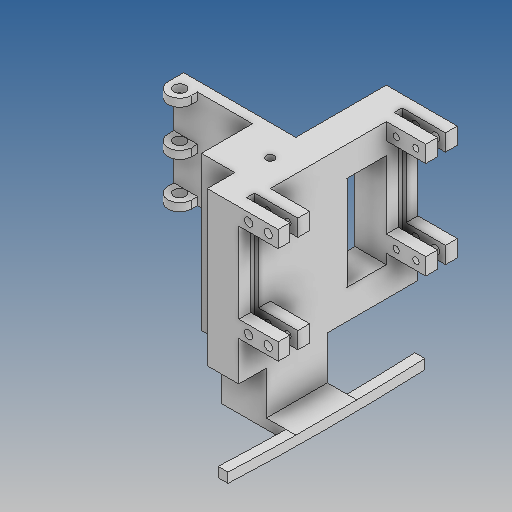
# Autodesk Inventor part: Korpus
Saved by Autodesk Inventor 2026.2 (Build 302298000, 298)
## iProperties
Created: 2025-08-31
Part Number: Korpus
Material: Generisch
Document SubType Name: Modeling
Designer: weyer
Density: 1 g/cm^3
Appearance: Vorgabe
Author: weyer
Autodesk Inventor part; units mm, degrees
sketch "Skizze1" plane through (0, 0, 0) normal (0, 0, 1) x (1, 0, 0)
  line L0 (-9.5, -10.5) -> (7.5, -10.5)
  line L1 (7.5, -10.5) -> (7.5, 10.5)
  line L2 (7.5, 10.5) -> (-9.5, 10.5)
  line L3 (-14.1, 0) -> (18.1, 0) projected
  line L4 (0, -21.7) -> (0, 21.7) projected
  line L5 (-9.5, -10.5) -> (-9.5, -15.5)
  line L6 (-9.5, -15.5) -> (13.5, -15.5)
  line L7 (-9.5, 10.5) -> (-9.5, 15.5)
  line L8 (-9.5, 15.5) -> (13.5, 15.5)
  line L9 (13.5, 15.5) -> (13.5, -15.5)
  point P0 (0, 0)
  dimension "d2" = 21
  dimension "d4" = 7.5
  dimension "d5" = 5
  dimension "d8" = 5
  dimension "d9" = 23
  dimension "d147" = 6
  dimension "d148" = 23
  constraints: 16 end point, 4 perpendicular, 2 vertical, 1 horizontal, 1 other
  measures "d2" distance between parallel lines of L0 L2
  measures "d4" distance between parallel lines of L1 L4
  measures "d5" distance of L0.start L5.end
  measures "d8" distance of L2.end L7.end
  measures "d9" distance of L7.end L8.end
  measures "d147" distance between parallel lines of L1 L9
  measures "d148" distance between parallel lines of L9 L5
extrude "Tower" add sketch "Skizze1" against normal blind 95 contours L0 L4 L6 L5 | L0 L1 L3 L9 L6 L4 | L1 L2 L4 L8 L9 L3 | L2 L7 L8 L4
ref_plane "Arbeitsebene1" through (0, 0, -95) normal (0, 0, -1) x (-1, 0, 0)
sketch "Skizze6" plane through (-9.5, 15.5, 0) normal (0, 1, 0) x (1, 0, 0)
  line L0 (23, 0) -> (23, 95) projected
  line L1 (23, 66.4131) -> (23, 0)
  line L2 (246, -7) -> (246, -5)
  line L3 (0, 0) -> (0, 95) projected
  line L4 (0, 0) -> (23, 0) projected
  line L5 (0, 0) -> (0, 95) projected
  line L6 (23, 95) -> (0, 95) projected
  line L7 (23, 0) -> (23, 95) projected
  line L8 (0, 0) -> (23, 0)
  line L9 (23, 0) -> (23, -10)
  line L10 (23, -10) -> (0, -10)
  line L11 (0, -10) -> (0, 0)
  dimension "d199" = 10
  constraints: 12 end point, 2 parallel, 1 horizontal, 1 perpendicular, 1 point on line, 1 vertical
  measures "d199" distance of L8.end L9.end
extrude "Gripperbogen" add sketch "Skizze6" against normal blind 31 contours L9 L10 L11 L4
sketch "Skizze12" plane through (0, 0, -95) normal (0, 0, -1) x (-1, 0, 0)
  line L0 (-214.5, 9.5) -> (-236.5, 9.5) projected
  line L1 (-236.5, 15.5) -> (-236.5, 9.5) projected
  line L2 (9.5, 15.5) -> (-236.5, 15.5) projected
  line L3 (9.5, 15.5) -> (9.5, -15.5) projected
  line L4 (-136.5, -15.5) -> (9.5, -15.5) projected
  line L5 (-136.5, -15.5) -> (-206.5, 0) projected
  line L6 (-206.5, 0) -> (-236.5, 0) projected
  line L7 (-236.5, 6) -> (-236.5, 0) projected
  line L8 (-236.5, 6) -> (-214.5, 6) projected
  line L9 (-214.5, 6) -> (-214.5, 9.5) projected
  line L10 (-7.5, 10.5) -> (9.5, 10.5) projected
  line L11 (9.5, 10.5) -> (9.5, 15.5) projected
  line L12 (9.5, 15.5) -> (-13.5, 15.5) projected
  line L13 (-13.5, 15.5) -> (-13.5, -15.5) projected
  line L14 (-13.5, -15.5) -> (9.5, -15.5) projected
  line L15 (9.5, -15.5) -> (9.5, -10.5) projected
  line L16 (9.5, -10.5) -> (-7.5, -10.5) projected
  line L17 (-7.5, -10.5) -> (-7.5, 10.5) projected
  line L18 (-13.5, 15.5) -> (-13.5, -15.5) projected
  line L19 (-13.5, -15.5) -> (9.5, -15.5)
  line L20 (9.5, -15.5) -> (9.5, 15.5)
  line L21 (9.5, 15.5) -> (-13.5, 15.5)
  line L22 (-13.5, 15.5) -> (-13.5, -15.5)
  point P0 (9.5, 25.25)
  point P1 (-13.5, -5.25)
  point P2 (-13.5, 15.5)
  constraints: 8 end point, 2 parallel, 1 horizontal, 1 perpendicular
extrude "Extrusion10" add sketch "Skizze12" against normal blind 10 contours L2 L3 L10 L17 L16 L4 L13 | L3 L16 L17 L10
ref_plane "Arbeitsebene3" through (0, 0, -113.5) normal (0, 0, -1) x (-1, 0, 0)
ref_plane "Arbeitsebene4" through (-9.5, -5.25, -113.5) normal (-1, 0, 0) x (0, 0, 1)
sketch "Skizze18" plane through (0, 0, -85) normal (0, 0, 1) x (1, 0, 0)
  line L0 (7.5, 10.5) -> (7.5, -10.5) projected
  line L1 (-9.5, 10.5) -> (7.5, 10.5) projected
  circle A0 centre (2, 0) radius 2.75
  line L2 (7.5, -10.5) -> (-9.5, -10.5) projected
  line L3 (-9.5, 10.5) -> (-9.5, -10.5) projected
  point P0 (0, 0)
  dimension "d132" = 5.5
  dimension "d154" = 0
  dimension "d155" = 11.5
  dimension "d161" = 21
  dimension "d162" = 17
  constraints: 1 centre point
  measures "d132" diameter of A0
  measures "d154" vertical distance of point (0, 0) A0.centre
  measures "d155" distance from line of L3 A0.centre
  measures "d161" distance between parallel lines of L2 L1
  measures "d162" distance between parallel lines of L0 L3
extrude "Extrusion15" cut sketch "Skizze18" against normal through all contours A0
sketch "Skizze19" plane through (-9.5, -15.5, -95) normal (-1, 0, 0) x (0, 0, 1)
  line L0 (0, 0) -> (0, 31) projected
  line L1 (95, 26) -> (10, 26) projected
  line L2 (95, 5) -> (10, 5) projected
  line L3 (27, 31) -> (27, 0)
  line L4 (10, 26) -> (10, 5) projected
  line L5 (10, 26) -> (0, 26)
  line L6 (10, 5) -> (0, 5)
  line L7 (95, 26) -> (105, 26)
  line L8 (10, 26) -> (10, 5) projected
  line L9 (105, 0) -> (0, 0) projected
  line L10 (105, 31) -> (105, 0) projected
  line L11 (0, 31) -> (105, 31) projected
  line L12 (95, 26) -> (95, 5) projected
  point P0 (95, 15.5)
  point P1 (23.5, 25.5)
  point P2 (23.5, 5)
  point P3 (27, 26)
  point P4 (27, 5)
  point P5 (20, 10.25)
  point P6 (27, 0)
  dimension "d201" = 78
  constraints: 8 end point, 2 perpendicular, 2 point on line, 1 other
  measures "d201" distance between parallel lines of L3 L10
extrude "Extrusion16" add sketch "Skizze19" along normal blind 10 contours L3 L2 L12 L7 L10 L9 | L3 L11 L10 L7 L1
sketch "Skizze15" plane through (-9.5, -15.5, -95) normal (0, -1, 0) x (1, 0, 0)
  line L0 (23, 0) -> (0, 0) projected
  circle A0 centre (-1, 43) radius 2.25
  circle A1 centre (-1, 83) radius 2.25
  line L1 (23, 0) -> (23, 105) projected
  line L2 (23, 105) -> (-10, 105) projected
  line L3 (0, 27) -> (0, 0) projected
  line L4 (-10, 27) -> (-10, 105) projected
  line L5 (0, 27) -> (-10, 27) projected
  point P0 (9.5, 95)
  dimension "d138" = 4.5
  dimension "d142" = 4.5
  dimension "d143" = 40
  dimension "d200" = 24
  dimension "d279" = 22
  constraints: 2 centre point, 1 vertical alignment
  measures "d138" diameter of A0
  measures "d142" diameter of A1
  measures "d143" distance of A1.centre A0.centre
  measures "d200" distance from line of L1 A1.centre
  measures "d279" distance from line of L2 A1.centre
extrude "Extrusion13" cut sketch "Skizze15" against normal blind 100 contours A0 | A1
sketch "Skizze35" plane through (13.5, -15.5, -95) normal (1, 0, 0) x (0, 0, -1)
  line L0 (-100, 31) -> (0, 31) projected
  line L1 (-100, 0) -> (0, 0) projected
  line L2 (0, 31) -> (0, 0) projected
  line L3 (0, 31) -> (0, 0) projected
  line L4 (0, 0) -> (-5, 0)
  line L5 (-5, 0) -> (-5, 31)
  line L6 (-5, 31) -> (0, 31)
  line L7 (0, 31) -> (0, 0)
  line L8 (-105, 31) -> (0, 31) projected
  line L9 (-105, 31) -> (-105, 0) projected
  line L10 (0, 0) -> (-105, 0) projected
  point P0 (-29.8382, 31)
  point P1 (-29.8382, 0)
  point P2 (-95, 15.5)
  point P3 (-5, 31)
  point P4 (-5, 0)
  point P5 (-80, 31)
  point P6 (-80, 0)
  dimension "d176" = 5
  constraints: 8 end point, 2 parallel, 1 horizontal, 1 perpendicular
  measures "d176" distance of L5.end L6.end
extrude "Extrusion22" add sketch "Skizze35" along normal blind 10 contours L0 L2 L1 L5
sketch "Skizze36" plane through (23.5, -15.5, -95) normal (1, 0, 0) x (0, 0, -1)
  line L0 (-5, 0) -> (0, 0) projected
  line L1 (0, 0) -> (0, 31) projected
  line L2 (0, 31) -> (-5, 31) projected
  line L3 (-5, 31) -> (-5, 0) projected
  arc A0 (-9.879, -89.9986) -> (-9.879, 121.0014) centre (-1120.404, 15.5014) ccw
  line L4 (-5, 15.5) -> (0, 15.5)
  arc A1 (-4.9014, -90.4715) -> (-4.9014, 121.4742) centre (-1120.404, 15.5014) ccw
  line L5 (-5, 15.5) -> (0, 15.5)
  line L6 (-14.7679, -34.5) -> (17.3967, -34.5)
  line L7 (-14.7679, 65.5) -> (14.0644, 65.5)
  point P0 (-95, 15.5)
  point P1 (-0.9951, 65.5)
  point P2 (-6.0001, 65.5)
  point P3 (-4.9867, 31)
  point P4 (-4.9867, 0)
  point P5 (-6.0002, -34.5)
  point P6 (-0.9952, -34.5)
  dimension "d181" = 5
  dimension "d182" = 100
  constraints: 8 end point, 4 point on circle, 3 horizontal, 2 centre point, 2 midpoint, 1 other
  measures "d181" radial gap between concentric circles of A0 A1
  measures "d182" distance between parallel lines of L7 L6
extrude "Extrusion23" add sketch "Skizze36" along normal blind 5
sketch "Skizze40" plane through (-19.5, -15.5, 10) normal (0, -1, 0) x (1, 0, 0)
  line L0 (33, -100) -> (33, 0) projected
  line L1 (33, 0) -> (0, 0) projected
  line L2 (33, 0) -> (17, 0)
  line L3 (17, 0) -> (17, -78)
  line L4 (17, -78) -> (33, -78)
  line L5 (33, -78) -> (33, 0)
  point P0 (19.5, -10)
  point P1 (17, 0)
  dimension "d202" = 16
  dimension "d203" = 78
  constraints: 8 end point, 2 parallel, 1 horizontal, 1 perpendicular
  measures "d202" distance of L4.end L3.end
  measures "d203" distance of L3.end L2.end
extrude "Extrusion26" add sketch "Skizze40" along normal blind 14
sketch "Skizze41" plane through (-19.5, 15.5, 10) normal (0, 1, 0) x (1, 0, 0)
  line L0 (0, 0) -> (33, 0) projected
  line L1 (33, 0) -> (33, 100) projected
  line L2 (33, 78) -> (33, 0) projected
  line L3 (33, 0) -> (17, 0) projected
  line L4 (17, 0) -> (17, 78) projected
  line L5 (17, 78) -> (33, 78) projected
  point P0 (19.5, 10)
  point P1 (33, 78)
extrude "Extrusion27" add sketch "Skizze41" along normal blind 46
sketch "Skizze42" plane through (13.5, -15.5, -90) normal (1, 0, 0) x (0, 0, -1)
  line L0 (-22, 31) -> (-22, 77) projected
  line L1 (-100, -14) -> (-100, 77) projected
  line L2 (-22, 0) -> (-22, -14) projected
  line L3 (-22, -4) -> (-100, -4)
  line L4 (-100, -4) -> (-100, -8)
  line L5 (-100, -8) -> (-22, -8)
  line L6 (-22, -8) -> (-22, -4)
  line L7 (-100, 77) -> (-22, 77) projected
  line L8 (-22, -14) -> (-100, -14) projected
  line L9 (-100, 71) -> (-22, 71)
  line L10 (-22, 71) -> (-22, 67)
  line L11 (-22, 67) -> (-100, 67)
  line L12 (-100, 67) -> (-100, 71)
  line L13 (-42, -14) -> (-42, 77)
  point P0 (-90, 15.5)
  point P1 (-22, -8)
  point P2 (-42, -8)
  point P3 (-42, -4)
  point P4 (-42, 67)
  point P5 (-42, 71)
  dimension "d209" = 4
  dimension "d241" = 6
  dimension "d242" = 4
  dimension "d243" = 6
  dimension "d268" = 58
  constraints: 18 end point, 6 point on line, 4 parallel, 3 perpendicular, 2 horizontal
  measures "d209" distance between parallel lines of L5 L3
  measures "d241" distance between parallel lines of L8 L5
  measures "d242" distance of L9.end L10.end
  measures "d243" distance between parallel lines of L7 L9
  measures "d268" distance between parallel lines of L13 L1
extrude "Extrusion28" cut sketch "Skizze42" against normal blind 2 contours L11 L1 L9 L13 | L13 L5 L1 L3
sketch "Skizze44" plane through (13.5, -15.5, -90) normal (1, 0, 0) x (0, 0, -1)
  line L0 (-100, -4) -> (-100, -8) projected
  line L1 (-100, -4) -> (-42, -4) projected
  line L2 (-22, 0) -> (-22, -14) projected
  line L3 (-42, -8) -> (-100, -8) projected
  line L4 (-100, -14) -> (-100, -8) projected
  line L5 (-22, -14) -> (-100, -14) projected
  line L6 (-22, 0) -> (-22, -14) projected
  line L7 (-22, 31) -> (-22, 77) projected
  line L8 (-100, 77) -> (-22, 77) projected
  line L9 (-100, 71) -> (-100, 77) projected
  line L10 (-100, -14) -> (-91.5, -14)
  line L11 (-91.5, -14) -> (-91.5, -8)
  line L12 (-91.5, -8) -> (-100, -8)
  line L13 (-100, -8) -> (-100, -14)
  line L14 (-50.5, -14) -> (-42, -14)
  line L15 (-42, -14) -> (-42, -8)
  line L16 (-42, -8) -> (-50.5, -8)
  line L17 (-50.5, -8) -> (-50.5, -14)
  line L18 (-22, -4) -> (-50.5, -4)
  line L19 (-50.5, -4) -> (-50.5, 2)
  line L20 (-50.5, 2) -> (-22, 2)
  line L21 (-22, 2) -> (-22, -4)
  line L22 (-100, -4) -> (-91.5, -4)
  line L23 (-91.5, -4) -> (-91.5, 2)
  line L24 (-91.5, 2) -> (-100, 2)
  line L25 (-100, 2) -> (-100, -4)
  line L26 (-100, -4) -> (-42, -4) projected
  line L27 (-22, 0) -> (-22, -14) projected
  line L28 (0, 0) -> (-22, 0) projected
  line L29 (0, 0) -> (0, 31) projected
  line L30 (-22, 31) -> (0, 31) projected
  line L31 (-42, -8) -> (-100, -8) projected
  line L32 (-100, -14) -> (-100, -8) projected
  line L33 (-22, -14) -> (-100, -14) projected
  line L34 (-42, 67) -> (-100, 67) projected
  line L35 (-100, -4) -> (-100, 67) projected
  line L36 (-100, 71) -> (-42, 71) projected
  line L37 (-91.5, 77) -> (-91.5, 71)
  line L38 (-100, 67) -> (-91.5, 67)
  line L39 (-91.5, 67) -> (-91.5, 61)
  line L40 (-91.5, 61) -> (-100, 61)
  line L41 (-100, 61) -> (-100, 67)
  line L42 (-50.5, 77) -> (-50.5, 71)
  line L43 (-22, 67) -> (-50.5, 67)
  line L44 (-50.5, 67) -> (-50.5, 61)
  line L45 (-50.5, 61) -> (-22, 61)
  line L46 (-22, 61) -> (-22, 67)
  line L47 (-42, -4) -> (-42, -8) projected
  line L48 (-42, 71) -> (-42, 67) projected
  line L49 (-100, -4) -> (-42, -4) projected
  line L50 (-42, -4) -> (-42, -8) projected
  line L51 (0, 0) -> (-22, 0) projected
  line L52 (0, 0) -> (0, 31) projected
  line L53 (-22, 31) -> (0, 31) projected
  line L54 (-22, 31) -> (-22, 77) projected
  line L55 (-100, 77) -> (-22, 77) projected
  line L56 (-100, 71) -> (-100, 77) projected
  line L57 (-100, 71) -> (-42, 71) projected
  line L58 (-42, 71) -> (-42, 67) projected
  line L59 (-42, 67) -> (-100, 67) projected
  line L60 (-100, -4) -> (-100, 67) projected
  line L61 (-100, 77) -> (-22, 77) projected
  line L62 (-42, -14) -> (-42, 77)
  point P0 (-90, 15.5)
  point P1 (-50.5, -11)
  point P2 (-50.5, -1)
  point P3 (-91.5, -11)
  point P4 (-91.5, -1)
  point P5 (-36.25, 2)
  point P6 (-95.75, 2)
  point P7 (-47, -2)
  point P8 (-100, 2)
  point P9 (-91.5, -4)
  point P10 (-91.5, 64)
  point P11 (-91.5, 74)
  point P12 (-50.5, 64)
  point P13 (-50.5, 74)
  point P14 (-100, 61)
  point P15 (-22, 0)
  point P16 (-42, -14)
  point P17 (-50.5, -4)
  point P18 (-100, 67)
  point P19 (-100, 61)
  point P20 (-100, 2)
  point P21 (-42, 61)
  point P22 (-42, 2)
  dimension "d216" = 8.5
  dimension "d217" = 8.5
  dimension "d218" = 41
  dimension "d219" = 6
  dimension "d244" = 6
  dimension "d245" = 6
  constraints: 54 end point, 12 parallel, 10 midpoint, 8 perpendicular, 8 point on line, 6 horizontal, 6 vertical alignment, 1 horizontal alignment, 1 vertical
  measures "d216" distance of L12.end L11.end
  measures "d217" distance of L16.end L15.end
  measures "d218" distance between parallel lines of L17 L11
  measures "d219" distance of L18.end L19.end
  measures "d244" distance of L38.end L39.end
  measures "d245" distance of L44.end L43.end
extrude "Extrusion29" add sketch "Skizze44" along normal blind 20 contours L25 L24 L23 L1 | L3 L11 L5 L4 | L19 L20 L62 L1 | L35 L34 L39 L40 | L3 L15 L5 L17 | L45 L44 L34 L62 | L36 L42 L8 L62 | L36 L9 L8 L37
sketch "Skizze45" plane through (-19.5, -29.5, 10) normal (0, -1, 0) x (1, 0, 0)
  line L0 (53, 0) -> (53, -8.5) projected
  line L1 (17, 0) -> (17, -78) projected
  line L2 (53, 0) -> (53, -58) projected
  line L3 (33, -58) -> (33, -49.5) projected
  line L4 (53, -4.25) -> (17, -4.25)
  circle A0 centre (38, -53.75) radius 2.1
  circle A1 centre (48, -53.75) radius 2.1
  circle A2 centre (38, -4.25) radius 2.1
  circle A3 centre (48, -4.25) radius 2.1
  line L5 (33, -49.5) -> (33, -8.5) projected
  line L6 (53, -53.75) -> (17, -53.75)
  point P0 (53, -78)
  point P1 (19.5, -10)
  point P2 (33, -53.75)
  dimension "d227" = 4.2
  dimension "d228" = 4.2
  dimension "d229" = 4.2
  dimension "d230" = 4.2
  dimension "d231" = 5
  dimension "d237" = 5
  constraints: 5 point on line, 4 centre point, 4 end point, 2 horizontal alignment, 2 midpoint, 2 perpendicular, 2 vertical alignment
  measures "d227" diameter of A0
  measures "d228" diameter of A1
  measures "d229" diameter of A2
  measures "d230" diameter of A3
  measures "d231" distance from line of L0 A3.centre
  measures "d237" distance from line of L5 A2.centre
extrude "Extrusion30" cut sketch "Skizze45" against normal blind 8 contours A3 L4 | L4 A3 | L6 A1 | A1 L6 | A2 L4 | L4 A2 | L6 A0 | A0 L6
sketch "Skizze46" plane through (-19.5, -15.5, -95) normal (-1, 0, 0) x (0, 0, 1)
  line L0 (27, 26) -> (95, 26) projected
  line L1 (105, 0) -> (105, 31) projected
  line L2 (105, 31) -> (27, 31) projected
  line L3 (27, 31) -> (27, 77) projected
  line L4 (105, -14) -> (27, -14) projected
  line L5 (27, 77) -> (27, -14)
  line L6 (95, 26) -> (105, 26)
  line L7 (55, 31) -> (55, 26)
  point P0 (95, 15.5)
  dimension "d267" = 50
  constraints: 6 end point, 3 point on line, 2 perpendicular, 1 vertical
  measures "d267" distance between parallel lines of L7 L1
extrude "Extrusion31" add sketch "Skizze46" along normal blind 40 contours L7 L2 L1 L6 L0
sketch "Skizze47" plane through (-19.5, -15.5, 10) normal (0, 0, 1) x (1, 0, 0)
  circle A0 centre (21.5, 15.5) radius 2.75 projected
  line L0 (27, 5) -> (10, 5) projected
  line L1 (27, 26) -> (27, 5) projected
  line L2 (10, 26) -> (27, 26) projected
  line L3 (10, 26) -> (10, 5) projected
  circle A1 centre (19.5, 15.5) radius 2.1
  point P0 (19.5, 15.5)
  dimension "d238" = 4.2
  constraints: 1 centre point, 1 coincident
  measures "d238" diameter of A1
extrude "Extrusion32" cut sketch "Skizze47" against normal blind 10 contours A1 A0 | A0 A1 picked at (19.7139, 15.5) picked at (18.3139, 15.5)
sketch "Skizze48" plane through (-19.5, 61.5, 10) normal (0, 1, 0) x (1, 0, 0)
  circle A0 centre (48, 4.25) radius 2.1 projected
  circle A1 centre (38, 4.25) radius 2.1 projected
  circle A2 centre (38, 53.75) radius 2.1 projected
  circle A3 centre (48, 53.75) radius 2.1 projected
  point P0 (19.5, 10)
extrude "Extrusion33" cut sketch "Skizze48" against normal blind 8
sketch "Skizze50" plane through (13.5, -13.5, -39.5) normal (0, 1, 0) x (1, 0, 0)
  line L0 (0, -49.5) -> (0, -41) projected
  line L1 (0, -49.5) -> (20, -49.5) projected
  line L2 (20, -41) -> (20, -49.5) projected
  line L3 (0, -41) -> (20, -41) projected
  circle A0 centre (15, -45.25) radius 2.1 projected
  circle A1 centre (5, -45.25) radius 2.1 projected
  circle A2 centre (5, 4.25) radius 2.1 projected
  circle A3 centre (15, 4.25) radius 2.1 projected
  circle A4 centre (15, -45.25) radius 2.1 projected
  circle A5 centre (15, -45.25) radius 1.6
  circle A6 centre (5, -45.25) radius 1.6
  circle A7 centre (15, 4.25) radius 1.6
  circle A8 centre (5, 4.25) radius 1.6
  point P0 (-13.5, -39.5)
  dimension "d248" = 3.2
  dimension "d249" = 3.2
  dimension "d250" = 3.2
  dimension "d251" = 3.2
  constraints: 4 centre point, 4 coincident
  measures "d248" diameter of A5
  measures "d249" diameter of A6
  measures "d250" diameter of A7
  measures "d251" diameter of A8
extrude "Extrusion34" cut sketch "Skizze50" against normal blind 8 contours A5 | A6 | A7 | A8
sketch "Skizze51" plane through (13.5, 45.5, 1.5) normal (0, -1, 0) x (1, 0, 0)
  line L0 (0, -49.5) -> (0, -41) projected
  line L1 (20, -41) -> (20, -49.5) projected
  line L2 (0, -41) -> (20, -41) projected
  circle A0 centre (5, -45.25) radius 1.6 projected
  circle A1 centre (15, -45.25) radius 1.6 projected
  circle A2 centre (5, 4.25) radius 1.6 projected
  circle A3 centre (15, 4.25) radius 1.6 projected
  line L3 (0, -49.5) -> (20, -49.5) projected
  point P0 (-13.5, -1.5)
extrude "Extrusion35" cut sketch "Skizze51" against normal blind 8 contours A0 | A1 | A2 | A3
sketch "Skizze55" plane through (-9.5, 10.5, -85) normal (0, -1, 0) x (1, 0, 0)
  line L0 (-10, 95) -> (-50, 95) projected
  line L1 (-50, 45) -> (-50, 95) projected
  line L2 (-10, 45) -> (-50, 45) projected
  line L3 (-38, 95) -> (-38, 45)
  line L4 (-50, 95) -> (-38, 95)
  line L5 (-38, 95) -> (-38, 91)
  line L6 (-38, 91) -> (-50, 91)
  line L7 (-50, 91) -> (-50, 95)
  line L8 (-50, 70) -> (-10, 70)
  line L9 (-50, 72) -> (-38, 72)
  line L10 (-38, 72) -> (-38, 68)
  line L11 (-38, 68) -> (-50, 68)
  line L12 (-50, 68) -> (-50, 72)
  line L13 (-50, 45) -> (-38, 45)
  line L14 (-38, 45) -> (-38, 49)
  line L15 (-38, 49) -> (-50, 49)
  line L16 (-50, 49) -> (-50, 45)
  point P0 (9.5, 85)
  point P1 (-50, 49)
  point P2 (-50, 68)
  dimension "d269" = 12
  dimension "d270" = 4
  dimension "d271" = 4
  dimension "d272" = 4
  constraints: 28 end point, 6 parallel, 6 point on line, 4 horizontal, 4 perpendicular, 1 midpoint, 1 other
  measures "d269" distance between parallel lines of L1 L3
  measures "d270" distance of L4.end L5.end
  measures "d271" distance of L9.end L10.end
  measures "d272" distance of L14.end L13.end
extrude "Extrusion39" add sketch "Skizze55" along normal blind 9 contours L3 L6 L1 L0 | L3 L8 L1 L9 | L3 L11 L1 L8 | L3 L2 L1 L15
sketch "Skizze56" plane through (-19.5, -15.5, 10) normal (0, 0, 1) x (1, 0, 0)
  line L0 (-40, 31) -> (-40, 17) projected
  line L1 (-28, 17) -> (-40, 17) projected
  line L2 (-28, 26) -> (-28, 17) projected
  line L3 (-28, 26) -> (-40, 26)
  line L4 (-34, 26) -> (-34, 17)
  circle A0 centre (-34, 23) radius 3
  arc A1 (-40, 23) -> (-28, 23) centre (-34, 23) ccw
  point P0 (-34, 17)
  dimension "d275" = 6
  dimension "d276" = 3
  constraints: 4 end point, 4 point on line, 2 centre point, 2 midpoint, 2 point on circle, 1 coincident, 1 perpendicular, 1 tangent
  measures "d275" diameter of A0
  measures "d276" distance from line of A0.centre L3
extrude "Extrusion40" cut sketch "Skizze56" against normal blind 80 contours A1 L1 L0 | A0 L4 | L4 A0 | A1 L2 L1
sketch "Skizze57" plane through (13.5, -15.5, -90) normal (1, 0, 0) x (0, 0, -1)
  line L0 (-100, 2) -> (-100, 61) projected
  line L1 (-22, 31) -> (-22, 77) projected
  line L2 (-42, 61) -> (-50.5, 61) projected
  line L3 (-85, 61) -> (-37, 61)
  line L4 (-37, 61) -> (-37, 41)
  line L5 (-37, 41) -> (-85, 41)
  line L6 (-85, 41) -> (-85, 61)
  line L7 (-100, 61) -> (-91.5, 61) projected
  point P0 (-90, 15.5)
  point P1 (-95.75, 61)
  point P2 (-61, 61)
  dimension "d280" = 20
  dimension "d281" = 15
  dimension "d282" = 15
  constraints: 8 end point, 2 midpoint, 2 parallel, 1 horizontal, 1 horizontal alignment, 1 perpendicular
  measures "d280" distance of L3.end L4.end
  measures "d281" distance between parallel lines of L0 L6
  measures "d282" distance between parallel lines of L1 L4
extrude "Extrusion41" cut sketch "Skizze57" against normal blind 80
